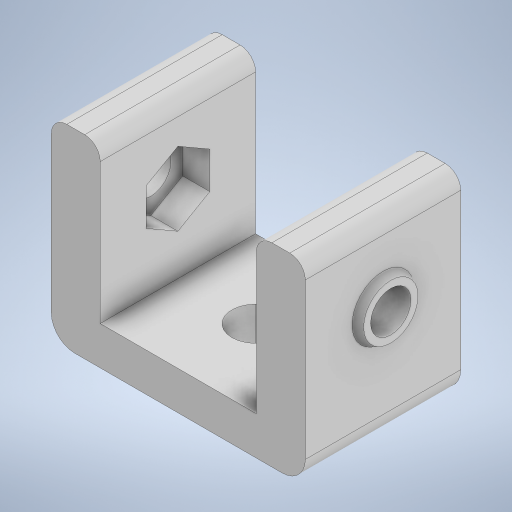
# Autodesk Inventor part: Idle Bearing mount2
Saved by Autodesk Inventor 2023.1 (Build 271208000, 208)
## iProperties
Created: 2022-10-30
Part Number: Idle Bearing mount2
Material: Generic
Document SubType Name: Modeling
Designer: nicol
Density: 1 g/cm^3
Appearance: Default
Author: nicol
Autodesk Inventor part; units mm, degrees
ref_plane "YZ Plane" through (0, 0, 0) normal (1, 0, 0) x (0, 1, 0)
ref_plane "XZ Plane" through (0, 0, 0) normal (0, 1, 0) x (-1, 0, 0)
ref_plane "XY Plane" through (0, 0, 0) normal (0, 0, 1) x (1, 0, 0)
sketch "Sketch1" plane through (0, 0, 0) normal (0, 0, 1) x (1, 0, 0)
  line L0 (0, 0) -> (0, 25)
  line L1 (0, 25) -> (6.35, 25)
  line L2 (6.35, 25) -> (6.35, 5)
  line L3 (6.35, 5) -> (26.35, 5)
  line L4 (26.35, 5) -> (26.35, 25)
  line L5 (26.35, 25) -> (32.7, 25)
  line L6 (32.7, 25) -> (32.7, 0)
  line L7 (32.7, 0) -> (0, 0)
  dimension "d0" = 20
  dimension "d1" = 6.35
  dimension "d2" = 20
  dimension "d3" = 5
  constraints: 16 end point, 7 perpendicular, 2 collinear, 1 vertical
  measures "d0" distance of L2.end L3.end
  measures "d1" distance of L0.end L1.end
  measures "d2" distance of L1.end L2.end
  measures "d3" distance between parallel lines of L7 L3
extrude "Extrusion1" add sketch "Sketch1" along normal blind 20
thicken "Thicken1" operation add thickness 0.05 both sides no extend neighbours yes toward (-1, 0, 0) faces at (6.35, 11.6667, 6.6667) (19.6833, 5, 6.6667) (26.35, 18.3333, 6.6667)
sketch "Sketch2" plane through (6.3, 4.95, 0) normal (0, 1, 0) x (1, 0, 0)
  line L0 (20.1, 0) -> (0, 0) projected
  line L1 (0, 0) -> (0, -20) projected
  line L2 (20.1, -20) -> (0, -20) projected
  line L3 (20.1, 0) -> (20.1, -20) projected
  line L4 (10.05, -6.7668) -> (12.85, -8.3834)
  line L5 (12.85, -8.3834) -> (12.85, -11.6166)
  line L6 (12.85, -11.6166) -> (10.05, -13.2332)
  line L7 (10.05, -13.2332) -> (7.25, -11.6166)
  line L8 (7.25, -11.6166) -> (7.25, -8.3834)
  line L9 (7.25, -8.3834) -> (10.05, -6.7668)
  line L10 (0, 0) -> (0, -20) projected
  point P0 (-6.3, 0)
  point P1 (10.05, -10)
  point P2 (0, -10)
  point P3 (10.05, -20)
  dimension "d8" = 5.6
  constraints: 12 end point, 2 midpoint, 1 horizontal alignment, 1 vertical, 1 vertical alignment, 13 other
  measures "d8" distance between parallel lines of L5 L8
hole "Hole1" at (16.35, 4.95, 10) direction (0, -1, 0) diameter 6.2 end through all
fillet "Fillet1" radius 3 2 edges at (0, 0, 10) (32.7, 0, 10)
sketch "Sketch3" plane through (26.4, 4.95, 0) normal (-1, 0, 0) x (0, 0, 1)
  line L0 (0, 20.05) -> (0, 0) projected
  line L1 (0, 0) -> (20, 0) projected
  line L2 (20, 20.05) -> (20, 0) projected
  line L3 (0, 20.05) -> (20, 20.05) projected
  line L4 (5.9, 12.3921) -> (10, 14.7593)
  line L5 (10, 14.7593) -> (14.1, 12.3921)
  line L6 (14.1, 12.3921) -> (14.1, 7.6579)
  line L7 (14.1, 7.6579) -> (10, 5.2907)
  line L8 (10, 5.2907) -> (5.9, 7.6579)
  line L9 (5.9, 7.6579) -> (5.9, 12.3921)
  point P0 (0, -4.95)
  point P1 (10, 10.025)
  point P2 (10, 20.05)
  point P3 (20, 10.025)
  dimension "d19" = 8.2
  constraints: 12 end point, 2 midpoint, 1 horizontal alignment, 1 vertical, 1 vertical alignment, 13 other
  measures "d19" distance between parallel lines of L6 L9
extrude "Extrusion3" cut sketch "Sketch3" against normal blind 3.5 contours L4 L5 L6 L7 L8 L9
hole "Hole2" at (26.4, 14.975, 10) direction (1, 0, 0) diameter 5.2 end through all
sketch "Sketch4" plane through (32.7, 25, 20) normal (1, 0, 0) x (0, 0, -1)
  circle A0 centre (10, -10.025) radius 2.6 projected
  circle A1 centre (10, -10.025) radius 3.5
  point P0 (20, -25)
  dimension "d29" = 7
  constraints: 1 centre point, 1 coincident
  measures "d29" diameter of A1
extrude "Extrusion4" add sketch "Sketch4" along normal blind 1
chamfer "Chamfer2" distance 0.5 distance2 1 1 edges at (32.7, 14.975, 13.5) measured on face at (32.7, 14.975, 14)
ref_plane "Work Plane1" through (16.35, 4.95, 0) normal (1, 0, 0) x (0, 0, -1)
mirror "Mirror1" about plane through (16.35, 4.95, 0) normal (1, 0, 0) of "Extrusion3", "Hole2", "Extrusion4"
fillet "Fillet2" radius 2 4 edges at (26.4, 25, 10) (32.7, 25, 10) (0, 25, 10) (6.3, 25, 10)
sketch "Sketch5" plane through (3, 0, 0) normal (0, -1, 0) x (1, 0, 0)
  line L0 (26.7, 20) -> (26.7, 0) projected
  line L1 (0, 20) -> (26.7, 20) projected
  line L2 (0, 0) -> (0, 20) projected
  line L3 (0, 0) -> (26.7, 0) projected
  circle A0 centre (13.35, 10) radius 3.1 projected
  line L4 (13.35, 14.3841) -> (17.7341, 10)
  line L5 (17.7341, 10) -> (13.35, 5.6159)
  line L6 (13.35, 5.6159) -> (8.9659, 10)
  line L7 (8.9659, 10) -> (13.35, 14.3841)
  line L8 (13.35, 14.3841) -> (13.35, 5.6159) construction
  line L9 (17.7341, 10) -> (8.9659, 10) construction
  circle A1 centre (13.35, 10) radius 3.1 projected
  point P0 (-3, 0)
  point P1 (11.158, 7.808)
  point P2 (15.542, 7.808)
  constraints: 12 end point, 2 midpoint, 2 parallel, 2 tangent, 1 perpendicular, 1 vertical
extrude "Extrusion5" cut sketch "Sketch5" against normal through all contours L5 L6 A0
chamfer "Chamfer3" distance 0.5 distance2 1 1 edges at (0, 14.975, 13.5) measured on face at (0, 14.975, 14)
body "Solid1"
